Autodesk Inventor part; units mm, degrees
(part 2 of 3)
  line L340 (105.027388, 41.472612) -> (145.027388, 41.472612) construction
  arc A224 (108.377388, 44.822612) -> (108.377388, 38.122612) centre (108.377388, 41.472612) ccw
  arc A225 (91.677388, 38.122612) -> (91.677388, 44.822612) centre (91.677388, 41.472612) ccw
  arc A226 (-58.322612, 38.122612) -> (-58.322612, 44.822612) centre (-58.322612, 41.472612) ccw
  line L341 (-91.622612, 38.122612) -> (-58.322612, 38.122612)
  line L342 (-58.322612, 44.822612) -> (-91.622612, 44.822612)
  line L343 (-94.972612, 41.472612) -> (-54.972612, 41.472612) construction
  arc A227 (-91.622612, 44.822612) -> (-91.622612, 38.122612) centre (-91.622612, 41.472612) ccw
  arc A228 (-41.622612, 34.822612) -> (-41.622612, 28.122612) centre (-41.622612, 31.472612) ccw
  line L344 (-41.622612, 28.122612) -> (-8.322612, 28.122612)
  line L345 (-8.322612, 34.822612) -> (-41.622612, 34.822612)
  line L346 (-44.972612, 31.472612) -> (-4.972612, 31.472612) construction
  arc A229 (-8.322612, 28.122612) -> (-8.322612, 34.822612) centre (-8.322612, 31.472612) ccw
  arc A230 (8.377388, 34.822612) -> (8.377388, 28.122612) centre (8.377388, 31.472612) ccw
  line L347 (8.377388, 28.122612) -> (41.677388, 28.122612)
  line L348 (41.677388, 34.822612) -> (8.377388, 34.822612)
  line L349 (5.027388, 31.472612) -> (45.027388, 31.472612) construction
  arc A231 (58.377388, 34.822612) -> (58.377388, 28.122612) centre (58.377388, 31.472612) ccw
  line L350 (58.377388, 28.122612) -> (91.677388, 28.122612)
  line L351 (91.677388, 34.822612) -> (58.377388, 34.822612)
  line L352 (55.027388, 31.472612) -> (95.027388, 31.472612) construction
  arc A232 (41.677388, 28.122612) -> (41.677388, 34.822612) centre (41.677388, 31.472612) ccw
  arc A233 (158.377388, 34.822612) -> (158.377388, 28.122612) centre (158.377388, 31.472612) ccw
  line L353 (158.377388, 28.122612) -> (191.677388, 28.122612)
  line L354 (191.677388, 34.822612) -> (158.377388, 34.822612)
  line L355 (155.027388, 31.472612) -> (195.027388, 31.472612) construction
  arc A234 (191.677388, 28.122612) -> (191.677388, 34.822612) centre (191.677388, 31.472612) ccw
  arc A235 (141.677388, 28.122612) -> (141.677388, 34.822612) centre (141.677388, 31.472612) ccw
  line L356 (108.377388, 28.122612) -> (141.677388, 28.122612)
  line L357 (141.677388, 34.822612) -> (108.377388, 34.822612)
  line L358 (105.027388, 31.472612) -> (145.027388, 31.472612) construction
  arc A236 (108.377388, 34.822612) -> (108.377388, 28.122612) centre (108.377388, 31.472612) ccw
  arc A237 (91.677388, 28.122612) -> (91.677388, 34.822612) centre (91.677388, 31.472612) ccw
  arc A238 (-58.322612, 28.122612) -> (-58.322612, 34.822612) centre (-58.322612, 31.472612) ccw
  line L359 (-91.622612, 28.122612) -> (-58.322612, 28.122612)
  line L360 (-58.322612, 34.822612) -> (-91.622612, 34.822612)
  line L361 (-94.972612, 31.472612) -> (-54.972612, 31.472612) construction
  arc A239 (-91.622612, 34.822612) -> (-91.622612, 28.122612) centre (-91.622612, 31.472612) ccw
  arc A240 (-41.622612, 24.822612) -> (-41.622612, 18.122612) centre (-41.622612, 21.472612) ccw
  line L362 (-41.622612, 18.122612) -> (-8.322612, 18.122612)
  line L363 (-8.322612, 24.822612) -> (-41.622612, 24.822612)
  line L364 (-44.972612, 21.472612) -> (-4.972612, 21.472612) construction
  arc A241 (-8.322612, 18.122612) -> (-8.322612, 24.822612) centre (-8.322612, 21.472612) ccw
  arc A242 (8.377388, 24.822612) -> (8.377388, 18.122612) centre (8.377388, 21.472612) ccw
  line L365 (8.377388, 18.122612) -> (41.677388, 18.122612)
  line L366 (41.677388, 24.822612) -> (8.377388, 24.822612)
  line L367 (5.027388, 21.472612) -> (45.027388, 21.472612) construction
  arc A243 (58.377388, 24.822612) -> (58.377388, 18.122612) centre (58.377388, 21.472612) ccw
  line L368 (58.377388, 18.122612) -> (91.677388, 18.122612)
  line L369 (91.677388, 24.822612) -> (58.377388, 24.822612)
  line L370 (55.027388, 21.472612) -> (95.027388, 21.472612) construction
  arc A244 (41.677388, 18.122612) -> (41.677388, 24.822612) centre (41.677388, 21.472612) ccw
  arc A245 (158.377388, 24.822612) -> (158.377388, 18.122612) centre (158.377388, 21.472612) ccw
  line L371 (158.377388, 18.122612) -> (191.677388, 18.122612)
  line L372 (191.677388, 24.822612) -> (158.377388, 24.822612)
  line L373 (155.027388, 21.472612) -> (195.027388, 21.472612) construction
  arc A246 (191.677388, 18.122612) -> (191.677388, 24.822612) centre (191.677388, 21.472612) ccw
  arc A247 (141.677388, 18.122612) -> (141.677388, 24.822612) centre (141.677388, 21.472612) ccw
  line L374 (108.377388, 18.122612) -> (141.677388, 18.122612)
  line L375 (141.677388, 24.822612) -> (108.377388, 24.822612)
  line L376 (105.027388, 21.472612) -> (145.027388, 21.472612) construction
  arc A248 (108.377388, 24.822612) -> (108.377388, 18.122612) centre (108.377388, 21.472612) ccw
  arc A249 (91.677388, 18.122612) -> (91.677388, 24.822612) centre (91.677388, 21.472612) ccw
  arc A250 (-58.322612, 18.122612) -> (-58.322612, 24.822612) centre (-58.322612, 21.472612) ccw
  line L377 (-91.622612, 18.122612) -> (-58.322612, 18.122612)
  line L378 (-58.322612, 24.822612) -> (-91.622612, 24.822612)
  line L379 (-94.972612, 21.472612) -> (-54.972612, 21.472612) construction
  arc A251 (-91.622612, 24.822612) -> (-91.622612, 18.122612) centre (-91.622612, 21.472612) ccw
  arc A252 (-41.622612, 14.822612) -> (-41.622612, 8.122612) centre (-41.622612, 11.472612) ccw
  line L380 (-41.622612, 8.122612) -> (-8.322612, 8.122612)
  line L381 (-8.322612, 14.822612) -> (-41.622612, 14.822612)
  line L382 (-44.972612, 11.472612) -> (-4.972612, 11.472612) construction
  arc A253 (-8.322612, 8.122612) -> (-8.322612, 14.822612) centre (-8.322612, 11.472612) ccw
  arc A254 (8.377388, 14.822612) -> (8.377388, 8.122612) centre (8.377388, 11.472612) ccw
  line L383 (8.377388, 8.122612) -> (41.677388, 8.122612)
  line L384 (41.677388, 14.822612) -> (8.377388, 14.822612)
  line L385 (5.027388, 11.472612) -> (45.027388, 11.472612) construction
  arc A255 (58.377388, 14.822612) -> (58.377388, 8.122612) centre (58.377388, 11.472612) ccw
  line L386 (58.377388, 8.122612) -> (91.677388, 8.122612)
  line L387 (91.677388, 14.822612) -> (58.377388, 14.822612)
  line L388 (55.027388, 11.472612) -> (95.027388, 11.472612) construction
  arc A256 (41.677388, 8.122612) -> (41.677388, 14.822612) centre (41.677388, 11.472612) ccw
  arc A257 (158.377388, 14.822612) -> (158.377388, 8.122612) centre (158.377388, 11.472612) ccw
  line L389 (158.377388, 8.122612) -> (191.677388, 8.122612)
  line L390 (191.677388, 14.822612) -> (158.377388, 14.822612)
  line L391 (155.027388, 11.472612) -> (195.027388, 11.472612) construction
  arc A258 (191.677388, 8.122612) -> (191.677388, 14.822612) centre (191.677388, 11.472612) ccw
  arc A259 (141.677388, 8.122612) -> (141.677388, 14.822612) centre (141.677388, 11.472612) ccw
  line L392 (108.377388, 8.122612) -> (141.677388, 8.122612)
  line L393 (141.677388, 14.822612) -> (108.377388, 14.822612)
  line L394 (105.027388, 11.472612) -> (145.027388, 11.472612) construction
  arc A260 (108.377388, 14.822612) -> (108.377388, 8.122612) centre (108.377388, 11.472612) ccw
  arc A261 (91.677388, 8.122612) -> (91.677388, 14.822612) centre (91.677388, 11.472612) ccw
  arc A262 (-58.322612, 8.122612) -> (-58.322612, 14.822612) centre (-58.322612, 11.472612) ccw
  line L395 (-91.622612, 8.122612) -> (-58.322612, 8.122612)
  line L396 (-58.322612, 14.822612) -> (-91.622612, 14.822612)
  line L397 (-94.972612, 11.472612) -> (-54.972612, 11.472612) construction
  arc A263 (-91.622612, 14.822612) -> (-91.622612, 8.122612) centre (-91.622612, 11.472612) ccw
  arc A264 (-41.622612, 4.822612) -> (-41.622612, -1.877388) centre (-41.622612, 1.472612) ccw
  line L398 (-41.622612, -1.877388) -> (-8.322612, -1.877388)
  line L399 (-8.322612, 4.822612) -> (-41.622612, 4.822612)
  line L400 (-44.972612, 1.472612) -> (-4.972612, 1.472612) construction
  arc A265 (-8.322612, -1.877388) -> (-8.322612, 4.822612) centre (-8.322612, 1.472612) ccw
  arc A266 (8.377388, 4.822612) -> (8.377388, -1.877388) centre (8.377388, 1.472612) ccw
  line L401 (8.377388, -1.877388) -> (41.677388, -1.877388)
  line L402 (41.677388, 4.822612) -> (8.377388, 4.822612)
  line L403 (5.027388, 1.472612) -> (45.027388, 1.472612) construction
  arc A267 (58.377388, 4.822612) -> (58.377388, -1.877388) centre (58.377388, 1.472612) ccw
  line L404 (58.377388, -1.877388) -> (91.677388, -1.877388)
  line L405 (91.677388, 4.822612) -> (58.377388, 4.822612)
  line L406 (55.027388, 1.472612) -> (95.027388, 1.472612) construction
  arc A268 (41.677388, -1.877388) -> (41.677388, 4.822612) centre (41.677388, 1.472612) ccw
  arc A269 (158.377388, 4.822612) -> (158.377388, -1.877388) centre (158.377388, 1.472612) ccw
  line L407 (158.377388, -1.877388) -> (191.677388, -1.877388)
  line L408 (191.677388, 4.822612) -> (158.377388, 4.822612)
  line L409 (155.027388, 1.472612) -> (195.027388, 1.472612) construction
  arc A270 (191.677388, -1.877388) -> (191.677388, 4.822612) centre (191.677388, 1.472612) ccw
  arc A271 (141.677388, -1.877388) -> (141.677388, 4.822612) centre (141.677388, 1.472612) ccw
  line L410 (108.377388, -1.877388) -> (141.677388, -1.877388)
  line L411 (141.677388, 4.822612) -> (108.377388, 4.822612)
  line L412 (105.027388, 1.472612) -> (145.027388, 1.472612) construction
  arc A272 (108.377388, 4.822612) -> (108.377388, -1.877388) centre (108.377388, 1.472612) ccw
  arc A273 (91.677388, -1.877388) -> (91.677388, 4.822612) centre (91.677388, 1.472612) ccw
  arc A274 (-58.322612, -1.877388) -> (-58.322612, 4.822612) centre (-58.322612, 1.472612) ccw
  line L413 (-91.622612, -1.877388) -> (-58.322612, -1.877388)
  line L414 (-58.322612, 4.822612) -> (-91.622612, 4.822612)
  line L415 (-94.972612, 1.472612) -> (-54.972612, 1.472612) construction
  arc A275 (-91.622612, 4.822612) -> (-91.622612, -1.877388) centre (-91.622612, 1.472612) ccw
  arc A276 (-41.622612, -5.177388) -> (-41.622612, -11.877388) centre (-41.622612, -8.527388) ccw
  line L416 (-41.622612, -11.877388) -> (-8.322612, -11.877388)
  line L417 (-8.322612, -5.177388) -> (-41.622612, -5.177388)
  line L418 (-44.972612, -8.527388) -> (-4.972612, -8.527388) construction
  arc A277 (-8.322612, -11.877388) -> (-8.322612, -5.177388) centre (-8.322612, -8.527388) ccw
  arc A278 (8.377388, -5.177388) -> (8.377388, -11.877388) centre (8.377388, -8.527388) ccw
  line L419 (8.377388, -11.877388) -> (41.677388, -11.877388)
  line L420 (41.677388, -5.177388) -> (8.377388, -5.177388)
  line L421 (5.027388, -8.527388) -> (45.027388, -8.527388) construction
  arc A279 (58.377388, -5.177388) -> (58.377388, -11.877388) centre (58.377388, -8.527388) ccw
  line L422 (58.377388, -11.877388) -> (91.677388, -11.877388)
  line L423 (91.677388, -5.177388) -> (58.377388, -5.177388)
  line L424 (55.027388, -8.527388) -> (95.027388, -8.527388) construction
  arc A280 (41.677388, -11.877388) -> (41.677388, -5.177388) centre (41.677388, -8.527388) ccw
  arc A281 (158.377388, -5.177388) -> (158.377388, -11.877388) centre (158.377388, -8.527388) ccw
  line L425 (158.377388, -11.877388) -> (191.677388, -11.877388)
  line L426 (191.677388, -5.177388) -> (158.377388, -5.177388)
  line L427 (155.027388, -8.527388) -> (195.027388, -8.527388) construction
  arc A282 (191.677388, -11.877388) -> (191.677388, -5.177388) centre (191.677388, -8.527388) ccw
  arc A283 (141.677388, -11.877388) -> (141.677388, -5.177388) centre (141.677388, -8.527388) ccw
  line L428 (108.377388, -11.877388) -> (141.677388, -11.877388)
  line L429 (141.677388, -5.177388) -> (108.377388, -5.177388)
  line L430 (105.027388, -8.527388) -> (145.027388, -8.527388) construction
  arc A284 (108.377388, -5.177388) -> (108.377388, -11.877388) centre (108.377388, -8.527388) ccw
  arc A285 (91.677388, -11.877388) -> (91.677388, -5.177388) centre (91.677388, -8.527388) ccw
  arc A286 (-58.322612, -11.877388) -> (-58.322612, -5.177388) centre (-58.322612, -8.527388) ccw
  line L431 (-91.622612, -11.877388) -> (-58.322612, -11.877388)
  line L432 (-58.322612, -5.177388) -> (-91.622612, -5.177388)
  line L433 (-94.972612, -8.527388) -> (-54.972612, -8.527388) construction
  arc A287 (-91.622612, -5.177388) -> (-91.622612, -11.877388) centre (-91.622612, -8.527388) ccw
  arc A288 (-41.622612, -15.177388) -> (-41.622612, -21.877388) centre (-41.622612, -18.527388) ccw
  line L434 (-41.622612, -21.877388) -> (-8.322612, -21.877388)
  line L435 (-8.322612, -15.177388) -> (-41.622612, -15.177388)
  line L436 (-44.972612, -18.527388) -> (-4.972612, -18.527388) construction
  arc A289 (-8.322612, -21.877388) -> (-8.322612, -15.177388) centre (-8.322612, -18.527388) ccw
  arc A290 (8.377388, -15.177388) -> (8.377388, -21.877388) centre (8.377388, -18.527388) ccw
  line L437 (8.377388, -21.877388) -> (41.677388, -21.877388)
  line L438 (41.677388, -15.177388) -> (8.377388, -15.177388)
  line L439 (5.027388, -18.527388) -> (45.027388, -18.527388) construction
  arc A291 (58.377388, -15.177388) -> (58.377388, -21.877388) centre (58.377388, -18.527388) ccw
  line L440 (58.377388, -21.877388) -> (91.677388, -21.877388)
  line L441 (91.677388, -15.177388) -> (58.377388, -15.177388)
  line L442 (55.027388, -18.527388) -> (95.027388, -18.527388) construction
  arc A292 (41.677388, -21.877388) -> (41.677388, -15.177388) centre (41.677388, -18.527388) ccw
  arc A293 (158.377388, -15.177388) -> (158.377388, -21.877388) centre (158.377388, -18.527388) ccw
  line L443 (158.377388, -21.877388) -> (191.677388, -21.877388)
  line L444 (191.677388, -15.177388) -> (158.377388, -15.177388)
  line L445 (155.027388, -18.527388) -> (195.027388, -18.527388) construction
  arc A294 (191.677388, -21.877388) -> (191.677388, -15.177388) centre (191.677388, -18.527388) ccw
  arc A295 (141.677388, -21.877388) -> (141.677388, -15.177388) centre (141.677388, -18.527388) ccw
  line L446 (108.377388, -21.877388) -> (141.677388, -21.877388)
  line L447 (141.677388, -15.177388) -> (108.377388, -15.177388)
  line L448 (105.027388, -18.527388) -> (145.027388, -18.527388) construction
  arc A296 (108.377388, -15.177388) -> (108.377388, -21.877388) centre (108.377388, -18.527388) ccw
  arc A297 (91.677388, -21.877388) -> (91.677388, -15.177388) centre (91.677388, -18.527388) ccw
  arc A298 (-58.322612, -21.877388) -> (-58.322612, -15.177388) centre (-58.322612, -18.527388) ccw
  line L449 (-91.622612, -21.877388) -> (-58.322612, -21.877388)
  line L450 (-58.322612, -15.177388) -> (-91.622612, -15.177388)
  line L451 (-94.972612, -18.527388) -> (-54.972612, -18.527388) construction
  arc A299 (-91.622612, -15.177388) -> (-91.622612, -21.877388) centre (-91.622612, -18.527388) ccw
  arc A300 (-41.622612, -25.177388) -> (-41.622612, -31.877388) centre (-41.622612, -28.527388) ccw
  line L452 (-41.622612, -31.877388) -> (-8.322612, -31.877388)
  line L453 (-8.322612, -25.177388) -> (-41.622612, -25.177388)
  line L454 (-44.972612, -28.527388) -> (-4.972612, -28.527388) construction
  arc A301 (-8.322612, -31.877388) -> (-8.322612, -25.177388) centre (-8.322612, -28.527388) ccw
  arc A302 (8.377388, -25.177388) -> (8.377388, -31.877388) centre (8.377388, -28.527388) ccw
  line L455 (8.377388, -31.877388) -> (41.677388, -31.877388)
  line L456 (41.677388, -25.177388) -> (8.377388, -25.177388)
  line L457 (5.027388, -28.527388) -> (45.027388, -28.527388) construction
  arc A303 (58.377388, -25.177388) -> (58.377388, -31.877388) centre (58.377388, -28.527388) ccw
  line L458 (58.377388, -31.877388) -> (91.677388, -31.877388)
  line L459 (91.677388, -25.177388) -> (58.377388, -25.177388)
  line L460 (55.027388, -28.527388) -> (95.027388, -28.527388) construction
  arc A304 (41.677388, -31.877388) -> (41.677388, -25.177388) centre (41.677388, -28.527388) ccw
  arc A305 (158.377388, -25.177388) -> (158.377388, -31.877388) centre (158.377388, -28.527388) ccw
  line L461 (158.377388, -31.877388) -> (191.677388, -31.877388)
  line L462 (191.677388, -25.177388) -> (158.377388, -25.177388)
  line L463 (155.027388, -28.527388) -> (195.027388, -28.527388) construction
  arc A306 (191.677388, -31.877388) -> (191.677388, -25.177388) centre (191.677388, -28.527388) ccw
  arc A307 (141.677388, -31.877388) -> (141.677388, -25.177388) centre (141.677388, -28.527388) ccw
  line L464 (108.377388, -31.877388) -> (141.677388, -31.877388)
  line L465 (141.677388, -25.177388) -> (108.377388, -25.177388)
  line L466 (105.027388, -28.527388) -> (145.027388, -28.527388) construction
  arc A308 (108.377388, -25.177388) -> (108.377388, -31.877388) centre (108.377388, -28.527388) ccw
  arc A309 (91.677388, -31.877388) -> (91.677388, -25.177388) centre (91.677388, -28.527388) ccw
  arc A310 (-58.322612, -31.877388) -> (-58.322612, -25.177388) centre (-58.322612, -28.527388) ccw
  line L467 (-91.622612, -31.877388) -> (-58.322612, -31.877388)
  line L468 (-58.322612, -25.177388) -> (-91.622612, -25.177388)
  line L469 (-94.972612, -28.527388) -> (-54.972612, -28.527388) construction
  arc A311 (-91.622612, -25.177388) -> (-91.622612, -31.877388) centre (-91.622612, -28.527388) ccw
  arc A312 (-41.622612, -35.177388) -> (-41.622612, -41.877388) centre (-41.622612, -38.527388) ccw
  line L470 (-41.622612, -41.877388) -> (-8.322612, -41.877388)
  line L471 (-8.322612, -35.177388) -> (-41.622612, -35.177388)
  line L472 (-44.972612, -38.527388) -> (-4.972612, -38.527388) construction
  arc A313 (-8.322612, -41.877388) -> (-8.322612, -35.177388) centre (-8.322612, -38.527388) ccw
  arc A314 (8.377388, -35.177388) -> (8.377388, -41.877388) centre (8.377388, -38.527388) ccw
  line L473 (8.377388, -41.877388) -> (41.677388, -41.877388)
  line L474 (41.677388, -35.177388) -> (8.377388, -35.177388)
  line L475 (5.027388, -38.527388) -> (45.027388, -38.527388) construction
  arc A315 (58.377388, -35.177388) -> (58.377388, -41.877388) centre (58.377388, -38.527388) ccw
  line L476 (58.377388, -41.877388) -> (91.677388, -41.877388)
  line L477 (91.677388, -35.177388) -> (58.377388, -35.177388)
  line L478 (55.027388, -38.527388) -> (95.027388, -38.527388) construction
  arc A316 (41.677388, -41.877388) -> (41.677388, -35.177388) centre (41.677388, -38.527388) ccw
  arc A317 (158.377388, -35.177388) -> (158.377388, -41.877388) centre (158.377388, -38.527388) ccw
  line L479 (158.377388, -41.877388) -> (191.677388, -41.877388)
  line L480 (191.677388, -35.177388) -> (158.377388, -35.177388)
  line L481 (155.027388, -38.527388) -> (195.027388, -38.527388) construction
  arc A318 (191.677388, -41.877388) -> (191.677388, -35.177388) centre (191.677388, -38.527388) ccw
  arc A319 (141.677388, -41.877388) -> (141.677388, -35.177388) centre (141.677388, -38.527388) ccw
  line L482 (108.377388, -41.877388) -> (141.677388, -41.877388)
  line L483 (141.677388, -35.177388) -> (108.377388, -35.177388)
  line L484 (105.027388, -38.527388) -> (145.027388, -38.527388) construction
  arc A320 (108.377388, -35.177388) -> (108.377388, -41.877388) centre (108.377388, -38.527388) ccw
  arc A321 (91.677388, -41.877388) -> (91.677388, -35.177388) centre (91.677388, -38.527388) ccw
  arc A322 (-58.322612, -41.877388) -> (-58.322612, -35.177388) centre (-58.322612, -38.527388) ccw
  line L485 (-91.622612, -41.877388) -> (-58.322612, -41.877388)
  line L486 (-58.322612, -35.177388) -> (-91.622612, -35.177388)
  line L487 (-94.972612, -38.527388) -> (-54.972612, -38.527388) construction
  arc A323 (-91.622612, -35.177388) -> (-91.622612, -41.877388) centre (-91.622612, -38.527388) ccw
  arc A324 (-41.622612, -45.177388) -> (-41.622612, -51.877388) centre (-41.622612, -48.527388) ccw
  line L488 (-41.622612, -51.877388) -> (-8.322612, -51.877388)
  line L489 (-8.322612, -45.177388) -> (-41.622612, -45.177388)
  line L490 (-44.972612, -48.527388) -> (-4.972612, -48.527388) construction
  arc A325 (-8.322612, -51.877388) -> (-8.322612, -45.177388) centre (-8.322612, -48.527388) ccw
  arc A326 (8.377388, -45.177388) -> (8.377388, -51.877388) centre (8.377388, -48.527388) ccw
  line L491 (8.377388, -51.877388) -> (41.677388, -51.877388)
  line L492 (41.677388, -45.177388) -> (8.377388, -45.177388)
  line L493 (5.027388, -48.527388) -> (45.027388, -48.527388) construction
  arc A327 (58.377388, -45.177388) -> (58.377388, -51.877388) centre (58.377388, -48.527388) ccw
  line L494 (58.377388, -51.877388) -> (91.677388, -51.877388)
  line L495 (91.677388, -45.177388) -> (58.377388, -45.177388)
  line L496 (55.027388, -48.527388) -> (95.027388, -48.527388) construction
  arc A328 (41.677388, -51.877388) -> (41.677388, -45.177388) centre (41.677388, -48.527388) ccw
  arc A329 (158.377388, -45.177388) -> (158.377388, -51.877388) centre (158.377388, -48.527388) ccw
  line L497 (158.377388, -51.877388) -> (191.677388, -51.877388)
  line L498 (191.677388, -45.177388) -> (158.377388, -45.177388)
  line L499 (155.027388, -48.527388) -> (195.027388, -48.527388) construction
  arc A330 (191.677388, -51.877388) -> (191.677388, -45.177388) centre (191.677388, -48.527388) ccw
  arc A331 (141.677388, -51.877388) -> (141.677388, -45.177388) centre (141.677388, -48.527388) ccw
  line L500 (108.377388, -51.877388) -> (141.677388, -51.877388)
  line L501 (141.677388, -45.177388) -> (108.377388, -45.177388)
  line L502 (105.027388, -48.527388) -> (145.027388, -48.527388) construction
  arc A332 (108.377388, -45.177388) -> (108.377388, -51.877388) centre (108.377388, -48.527388) ccw
  arc A333 (91.677388, -51.877388) -> (91.677388, -45.177388) centre (91.677388, -48.527388) ccw
  arc A334 (-58.322612, -51.877388) -> (-58.322612, -45.177388) centre (-58.322612, -48.527388) ccw
  line L503 (-91.622612, -51.877388) -> (-58.322612, -51.877388)
  line L504 (-58.322612, -45.177388) -> (-91.622612, -45.177388)
  line L505 (-94.972612, -48.527388) -> (-54.972612, -48.527388) construction
  arc A335 (-91.622612, -45.177388) -> (-91.622612, -51.877388) centre (-91.622612, -48.527388) ccw
  arc A336 (-41.622612, -55.177388) -> (-41.622612, -61.877388) centre (-41.622612, -58.527388) ccw
  line L506 (-41.622612, -61.877388) -> (-8.322612, -61.877388)
  line L507 (-8.322612, -55.177388) -> (-41.622612, -55.177388)
  line L508 (-44.972612, -58.527388) -> (-4.972612, -58.527388) construction
  arc A337 (-8.322612, -61.877388) -> (-8.322612, -55.177388) centre (-8.322612, -58.527388) ccw
  arc A338 (8.377388, -55.177388) -> (8.377388, -61.877388) centre (8.377388, -58.527388) ccw
  line L509 (8.377388, -61.877388) -> (41.677388, -61.877388)
  line L510 (41.677388, -55.177388) -> (8.377388, -55.177388)
  line L511 (5.027388, -58.527388) -> (45.027388, -58.527388) construction
  arc A339 (58.377388, -55.177388) -> (58.377388, -61.877388) centre (58.377388, -58.527388) ccw
  line L512 (58.377388, -61.877388) -> (91.677388, -61.877388)
  line L513 (91.677388, -55.177388) -> (58.377388, -55.177388)
  line L514 (55.027388, -58.527388) -> (95.027388, -58.527388) construction
  arc A340 (41.677388, -61.877388) -> (41.677388, -55.177388) centre (41.677388, -58.527388) ccw
  arc A341 (158.377388, -55.177388) -> (158.377388, -61.877388) centre (158.377388, -58.527388) ccw
  line L515 (158.377388, -61.877388) -> (191.677388, -61.877388)
  line L516 (191.677388, -55.177388) -> (158.377388, -55.177388)
  line L517 (155.027388, -58.527388) -> (195.027388, -58.527388) construction
  arc A342 (191.677388, -61.877388) -> (191.677388, -55.177388) centre (191.677388, -58.527388) ccw
  arc A343 (141.677388, -61.877388) -> (141.677388, -55.177388) centre (141.677388, -58.527388) ccw
  line L518 (108.377388, -61.877388) -> (141.677388, -61.877388)
  line L519 (141.677388, -55.177388) -> (108.377388, -55.177388)
  line L520 (105.027388, -58.527388) -> (145.027388, -58.527388) construction
  arc A344 (108.377388, -55.177388) -> (108.377388, -61.877388) centre (108.377388, -58.527388) ccw
  arc A345 (91.677388, -61.877388) -> (91.677388, -55.177388) centre (91.677388, -58.527388) ccw
  arc A346 (-58.322612, -61.877388) -> (-58.322612, -55.177388) centre (-58.322612, -58.527388) ccw
  line L521 (-91.622612, -61.877388) -> (-58.322612, -61.877388)
  line L522 (-58.322612, -55.177388) -> (-91.622612, -55.177388)
  line L523 (-94.972612, -58.527388) -> (-54.972612, -58.527388) construction
  arc A347 (-91.622612, -55.177388) -> (-91.622612, -61.877388) centre (-91.622612, -58.527388) ccw
  arc A348 (-41.622612, -65.177388) -> (-41.622612, -71.877388) centre (-41.622612, -68.527388) ccw
  line L524 (-41.622612, -71.877388) -> (-8.322612, -71.877388)
  line L525 (-8.322612, -65.177388) -> (-41.622612, -65.177388)
  line L526 (-44.972612, -68.527388) -> (-4.972612, -68.527388) construction
  arc A349 (-8.322612, -71.877388) -> (-8.322612, -65.177388) centre (-8.322612, -68.527388) ccw
  arc A350 (8.377388, -65.177388) -> (8.377388, -71.877388) centre (8.377388, -68.527388) ccw
  line L527 (8.377388, -71.877388) -> (41.677388, -71.877388)
  line L528 (41.677388, -65.177388) -> (8.377388, -65.177388)
  line L529 (5.027388, -68.527388) -> (45.027388, -68.527388) construction
  arc A351 (58.377388, -65.177388) -> (58.377388, -71.877388) centre (58.377388, -68.527388) ccw
  line L530 (58.377388, -71.877388) -> (91.677388, -71.877388)
  line L531 (91.677388, -65.177388) -> (58.377388, -65.177388)
  line L532 (55.027388, -68.527388) -> (95.027388, -68.527388) construction
  arc A352 (41.677388, -71.877388) -> (41.677388, -65.177388) centre (41.677388, -68.527388) ccw
  arc A353 (158.377388, -65.177388) -> (158.377388, -71.877388) centre (158.377388, -68.527388) ccw
  line L533 (158.377388, -71.877388) -> (191.677388, -71.877388)
  line L534 (191.677388, -65.177388) -> (158.377388, -65.177388)
  line L535 (155.027388, -68.527388) -> (195.027388, -68.527388) construction
  arc A354 (191.677388, -71.877388) -> (191.677388, -65.177388) centre (191.677388, -68.527388) ccw
  arc A355 (141.677388, -71.877388) -> (141.677388, -65.177388) centre (141.677388, -68.527388) ccw
  line L536 (108.377388, -71.877388) -> (141.677388, -71.877388)
  line L537 (141.677388, -65.177388) -> (108.377388, -65.177388)
  line L538 (105.027388, -68.527388) -> (145.027388, -68.527388) construction
  arc A356 (108.377388, -65.177388) -> (108.377388, -71.877388) centre (108.377388, -68.527388) ccw
  arc A357 (91.677388, -71.877388) -> (91.677388, -65.177388) centre (91.677388, -68.527388) ccw
  arc A358 (-58.322612, -71.877388) -> (-58.322612, -65.177388) centre (-58.322612, -68.527388) ccw
  line L539 (-91.622612, -71.877388) -> (-58.322612, -71.877388)
  line L540 (-58.322612, -65.177388) -> (-91.622612, -65.177388)
  line L541 (-94.972612, -68.527388) -> (-54.972612, -68.527388) construction
  arc A359 (-91.622612, -65.177388) -> (-91.622612, -71.877388) centre (-91.622612, -68.527388) ccw
  arc A360 (-41.622612, -75.177388) -> (-41.622612, -81.877388) centre (-41.622612, -78.527388) ccw
  line L542 (-41.622612, -81.877388) -> (-8.322612, -81.877388)
  line L543 (-8.322612, -75.177388) -> (-41.622612, -75.177388)
  line L544 (-44.972612, -78.527388) -> (-4.972612, -78.527388) construction
  arc A361 (-8.322612, -81.877388) -> (-8.322612, -75.177388) centre (-8.322612, -78.527388) ccw
  arc A362 (8.377388, -75.177388) -> (8.377388, -81.877388) centre (8.377388, -78.527388) ccw
  line L545 (8.377388, -81.877388) -> (41.677388, -81.877388)
  line L546 (41.677388, -75.177388) -> (8.377388, -75.177388)
  line L547 (5.027388, -78.527388) -> (45.027388, -78.527388) construction
  arc A363 (58.377388, -75.177388) -> (58.377388, -81.877388) centre (58.377388, -78.527388) ccw
  line L548 (58.377388, -81.877388) -> (91.677388, -81.877388)
  line L549 (91.677388, -75.177388) -> (58.377388, -75.177388)
  line L550 (55.027388, -78.527388) -> (95.027388, -78.527388) construction
  arc A364 (41.677388, -81.877388) -> (41.677388, -75.177388) centre (41.677388, -78.527388) ccw
  arc A365 (158.377388, -75.177388) -> (158.377388, -81.877388) centre (158.377388, -78.527388) ccw
  line L551 (158.377388, -81.877388) -> (191.677388, -81.877388)
  line L552 (191.677388, -75.177388) -> (158.377388, -75.177388)
  line L553 (155.027388, -78.527388) -> (195.027388, -78.527388) construction
  arc A366 (191.677388, -81.877388) -> (191.677388, -75.177388) centre (191.677388, -78.527388) ccw
  arc A367 (141.677388, -81.877388) -> (141.677388, -75.177388) centre (141.677388, -78.527388) ccw
  line L554 (108.377388, -81.877388) -> (141.677388, -81.877388)
  line L555 (141.677388, -75.177388) -> (108.377388, -75.177388)
  line L556 (105.027388, -78.527388) -> (145.027388, -78.527388) construction
  arc A368 (108.377388, -75.177388) -> (108.377388, -81.877388) centre (108.377388, -78.527388) ccw
  arc A369 (91.677388, -81.877388) -> (91.677388, -75.177388) centre (91.677388, -78.527388) ccw
  arc A370 (-58.322612, -81.877388) -> (-58.322612, -75.177388) centre (-58.322612, -78.527388) ccw
  line L557 (-91.622612, -81.877388) -> (-58.322612, -81.877388)
  line L558 (-58.322612, -75.177388) -> (-91.622612, -75.177388)
  line L559 (-94.972612, -78.527388) -> (-54.972612, -78.527388) construction
  arc A371 (-91.622612, -75.177388) -> (-91.622612, -81.877388) centre (-91.622612, -78.527388) ccw
  arc A372 (-41.622612, -85.177388) -> (-41.622612, -91.877388) centre (-41.622612, -88.527388) ccw
  line L560 (-41.622612, -91.877388) -> (-8.322612, -91.877388)
  line L561 (-8.322612, -85.177388) -> (-41.622612, -85.177388)
  line L562 (-44.972612, -88.527388) -> (-4.972612, -88.527388) construction
  arc A373 (-8.322612, -91.877388) -> (-8.322612, -85.177388) centre (-8.322612, -88.527388) ccw
  arc A374 (8.377388, -85.177388) -> (8.377388, -91.877388) centre (8.377388, -88.527388) ccw
  line L563 (8.377388, -91.877388) -> (41.677388, -91.877388)
  line L564 (41.677388, -85.177388) -> (8.377388, -85.177388)
  line L565 (5.027388, -88.527388) -> (45.027388, -88.527388) construction
  arc A375 (58.377388, -85.177388) -> (58.377388, -91.877388) centre (58.377388, -88.527388) ccw
  line L566 (58.377388, -91.877388) -> (91.677388, -91.877388)
  line L567 (91.677388, -85.177388) -> (58.377388, -85.177388)
  line L568 (55.027388, -88.527388) -> (95.027388, -88.527388) construction
  arc A376 (41.677388, -91.877388) -> (41.677388, -85.177388) centre (41.677388, -88.527388) ccw
  arc A377 (158.377388, -85.177388) -> (158.377388, -91.877388) centre (158.377388, -88.527388) ccw
  line L569 (158.377388, -91.877388) -> (191.677388, -91.877388)
  line L570 (191.677388, -85.177388) -> (158.377388, -85.177388)
  line L571 (155.027388, -88.527388) -> (195.027388, -88.527388) construction
  arc A378 (191.677388, -91.877388) -> (191.677388, -85.177388) centre (191.677388, -88.527388) ccw
  arc A379 (141.677388, -91.877388) -> (141.677388, -85.177388) centre (141.677388, -88.527388) ccw
  line L572 (108.377388, -91.877388) -> (141.677388, -91.877388)
  line L573 (141.677388, -85.177388) -> (108.377388, -85.177388)
  line L574 (105.027388, -88.527388) -> (145.027388, -88.527388) construction
  arc A380 (108.377388, -85.177388) -> (108.377388, -91.877388) centre (108.377388, -88.527388) ccw
  arc A381 (91.677388, -91.877388) -> (91.677388, -85.177388) centre (91.677388, -88.527388) ccw
  arc A382 (-58.322612, -91.877388) -> (-58.322612, -85.177388) centre (-58.322612, -88.527388) ccw
  line L575 (-91.622612, -91.877388) -> (-58.322612, -91.877388)
  line L576 (-58.322612, -85.177388) -> (-91.622612, -85.177388)
  line L577 (-94.972612, -88.527388) -> (-54.972612, -88.527388) construction
  arc A383 (-91.622612, -85.177388) -> (-91.622612, -91.877388) centre (-91.622612, -88.527388) ccw
  arc A384 (-41.622612, -95.177388) -> (-41.622612, -101.877388) centre (-41.622612, -98.527388) ccw
  line L578 (-41.622612, -101.877388) -> (-8.322612, -101.877388)
  line L579 (-8.322612, -95.177388) -> (-41.622612, -95.177388)
  line L580 (-44.972612, -98.527388) -> (-4.972612, -98.527388) construction
  arc A385 (-8.322612, -101.877388) -> (-8.322612, -95.177388) centre (-8.322612, -98.527388) ccw
  arc A386 (8.377388, -95.177388) -> (8.377388, -101.877388) centre (8.377388, -98.527388) ccw
  line L581 (8.377388, -101.877388) -> (41.677388, -101.877388)
  line L582 (41.677388, -95.177388) -> (8.377388, -95.177388)
  line L583 (5.027388, -98.527388) -> (45.027388, -98.527388) construction
  arc A387 (58.377388, -95.177388) -> (58.377388, -101.877388) centre (58.377388, -98.527388) ccw
  line L584 (58.377388, -101.877388) -> (91.677388, -101.877388)
  line L585 (91.677388, -95.177388) -> (58.377388, -95.177388)
  line L586 (55.027388, -98.527388) -> (95.027388, -98.527388) construction
  arc A388 (41.677388, -101.877388) -> (41.677388, -95.177388) centre (41.677388, -98.527388) ccw
  arc A389 (158.377388, -95.177388) -> (158.377388, -101.877388) centre (158.377388, -98.527388) ccw
  line L587 (158.377388, -101.877388) -> (191.677388, -101.877388)
  line L588 (191.677388, -95.177388) -> (158.377388, -95.177388)
  line L589 (155.027388, -98.527388) -> (195.027388, -98.527388) construction
  arc A390 (191.677388, -101.877388) -> (191.677388, -95.177388) centre (191.677388, -98.527388) ccw
  arc A391 (141.677388, -101.877388) -> (141.677388, -95.177388) centre (141.677388, -98.527388) ccw
  line L590 (108.377388, -101.877388) -> (141.677388, -101.877388)
  line L591 (141.677388, -95.177388) -> (108.377388, -95.177388)
  line L592 (105.027388, -98.527388) -> (145.027388, -98.527388) construction
  arc A392 (108.377388, -95.177388) -> (108.377388, -101.877388) centre (108.377388, -98.527388) ccw
  arc A393 (91.677388, -101.877388) -> (91.677388, -95.177388) centre (91.677388, -98.527388) ccw
  arc A394 (-58.322612, -101.877388) -> (-58.322612, -95.177388) centre (-58.322612, -98.527388) ccw
  line L593 (-91.622612, -101.877388) -> (-58.322612, -101.877388)
  line L594 (-58.322612, -95.177388) -> (-91.622612, -95.177388)
  line L595 (-94.972612, -98.527388) -> (-54.972612, -98.527388) construction
  arc A395 (-91.622612, -95.177388) -> (-91.622612, -101.877388) centre (-91.622612, -98.527388) ccw
  arc A396 (-41.622612, -105.177388) -> (-41.622612, -111.877388) centre (-41.622612, -108.527388) ccw
  line L596 (-41.622612, -111.877388) -> (-8.322612, -111.877388)
  line L597 (-8.322612, -105.177388) -> (-41.622612, -105.177388)
  line L598 (-44.972612, -108.527388) -> (-4.972612, -108.527388) construction
  arc A397 (-8.322612, -111.877388) -> (-8.322612, -105.177388) centre (-8.322612, -108.527388) ccw
  arc A398 (8.377388, -105.177388) -> (8.377388, -111.877388) centre (8.377388, -108.527388) ccw
  line L599 (8.377388, -111.877388) -> (41.677388, -111.877388)
  line L600 (41.677388, -105.177388) -> (8.377388, -105.177388)
  line L601 (5.027388, -108.527388) -> (45.027388, -108.527388) construction
  arc A399 (58.377388, -105.177388) -> (58.377388, -111.877388) centre (58.377388, -108.527388) ccw
  line L602 (58.377388, -111.877388) -> (91.677388, -111.877388)
  line L603 (91.677388, -105.177388) -> (58.377388, -105.177388)
  line L604 (55.027388, -108.527388) -> (95.027388, -108.527388) construction
  arc A400 (41.677388, -111.877388) -> (41.677388, -105.177388) centre (41.677388, -108.527388) ccw
  arc A401 (158.377388, -105.177388) -> (158.377388, -111.877388) centre (158.377388, -108.527388) ccw
  line L605 (158.377388, -111.877388) -> (191.677388, -111.877388)
  line L606 (191.677388, -105.177388) -> (158.377388, -105.177388)
  line L607 (155.027388, -108.527388) -> (195.027388, -108.527388) construction
  arc A402 (191.677388, -111.877388) -> (191.677388, -105.177388) centre (191.677388, -108.527388) ccw
  arc A403 (141.677388, -111.877388) -> (141.677388, -105.177388) centre (141.677388, -108.527388) ccw
  line L608 (108.377388, -111.877388) -> (141.677388, -111.877388)
  line L609 (141.677388, -105.177388) -> (108.377388, -105.177388)
  line L610 (105.027388, -108.527388) -> (145.027388, -108.527388) construction
  arc A404 (108.377388, -105.177388) -> (108.377388, -111.877388) centre (108.377388, -108.527388) ccw
  arc A405 (91.677388, -111.877388) -> (91.677388, -105.177388) centre (91.677388, -108.527388) ccw
  arc A406 (-58.322612, -111.877388) -> (-58.322612, -105.177388) centre (-58.322612, -108.527388) ccw
  line L611 (-91.622612, -111.877388) -> (-58.322612, -111.877388)
  line L612 (-58.322612, -105.177388) -> (-91.622612, -105.177388)
  line L613 (-94.972612, -108.527388) -> (-54.972612, -108.527388) construction
  arc A407 (-91.622612, -105.177388) -> (-91.622612, -111.877388) centre (-91.622612, -108.527388) ccw
  arc A408 (-41.622612, -115.177388) -> (-41.622612, -121.877388) centre (-41.622612, -118.527388) ccw
  line L614 (-41.622612, -121.877388) -> (-8.322612, -121.877388)
  line L615 (-8.322612, -115.177388) -> (-41.622612, -115.177388)
  line L616 (-44.972612, -118.527388) -> (-4.972612, -118.527388) construction
  arc A409 (-8.322612, -121.877388) -> (-8.322612, -115.177388) centre (-8.322612, -118.527388) ccw
  arc A410 (8.377388, -115.177388) -> (8.377388, -121.877388) centre (8.377388, -118.527388) ccw
  line L617 (8.377388, -121.877388) -> (41.677388, -121.877388)
  line L618 (41.677388, -115.177388) -> (8.377388, -115.177388)
  line L619 (5.027388, -118.527388) -> (45.027388, -118.527388) construction
  arc A411 (58.377388, -115.177388) -> (58.377388, -121.877388) centre (58.377388, -118.527388) ccw
  line L620 (58.377388, -121.877388) -> (91.677388, -121.877388)
  line L621 (91.677388, -115.177388) -> (58.377388, -115.177388)
  line L622 (55.027388, -118.527388) -> (95.027388, -118.527388) construction
  arc A412 (41.677388, -121.877388) -> (41.677388, -115.177388) centre (41.677388, -118.527388) ccw
  arc A413 (158.377388, -115.177388) -> (158.377388, -121.877388) centre (158.377388, -118.527388) ccw
  line L623 (158.377388, -121.877388) -> (191.677388, -121.877388)
  line L624 (191.677388, -115.177388) -> (158.377388, -115.177388)
  line L625 (155.027388, -118.527388) -> (195.027388, -118.527388) construction
  arc A414 (191.677388, -121.877388) -> (191.677388, -115.177388) centre (191.677388, -118.527388) ccw
  arc A415 (141.677388, -121.877388) -> (141.677388, -115.177388) centre (141.677388, -118.527388) ccw
  line L626 (108.377388, -121.877388) -> (141.677388, -121.877388)
  line L627 (141.677388, -115.177388) -> (108.377388, -115.177388)
  line L628 (105.027388, -118.527388) -> (145.027388, -118.527388) construction
  arc A416 (108.377388, -115.177388) -> (108.377388, -121.877388) centre (108.377388, -118.527388) ccw
  arc A417 (91.677388, -121.877388) -> (91.677388, -115.177388) centre (91.677388, -118.527388) ccw
  arc A418 (-58.322612, -121.877388) -> (-58.322612, -115.177388) centre (-58.322612, -118.527388) ccw
  line L629 (-91.622612, -121.877388) -> (-58.322612, -121.877388)
  line L630 (-58.322612, -115.177388) -> (-91.622612, -115.177388)
  line L631 (-94.972612, -118.527388) -> (-54.972612, -118.527388) construction
  arc A419 (-91.622612, -115.177388) -> (-91.622612, -121.877388) centre (-91.622612, -118.527388) ccw
  arc A420 (-41.622612, -125.177388) -> (-41.622612, -131.877388) centre (-41.622612, -128.527388) ccw
  line L632 (-41.622612, -131.877388) -> (-8.322612, -131.877388)
  line L633 (-8.322612, -125.177388) -> (-41.622612, -125.177388)
  line L634 (-44.972612, -128.527388) -> (-4.972612, -128.527388) construction
  arc A421 (-8.322612, -131.877388) -> (-8.322612, -125.177388) centre (-8.322612, -128.527388) ccw
  arc A422 (8.377388, -125.177388) -> (8.377388, -131.877388) centre (8.377388, -128.527388) ccw
  line L635 (8.377388, -131.877388) -> (41.677388, -131.877388)
  line L636 (41.677388, -125.177388) -> (8.377388, -125.177388)
  line L637 (5.027388, -128.527388) -> (45.027388, -128.527388) construction
  arc A423 (58.377388, -125.177388) -> (58.377388, -131.877388) centre (58.377388, -128.527388) ccw
  line L638 (58.377388, -131.877388) -> (91.677388, -131.877388)
  line L639 (91.677388, -125.177388) -> (58.377388, -125.177388)
  line L640 (55.027388, -128.527388) -> (95.027388, -128.527388) construction
  arc A424 (41.677388, -131.877388) -> (41.677388, -125.177388) centre (41.677388, -128.527388) ccw
  arc A425 (158.377388, -125.177388) -> (158.377388, -131.877388) centre (158.377388, -128.527388) ccw
  line L641 (158.377388, -131.877388) -> (191.677388, -131.877388)
  line L642 (191.677388, -125.177388) -> (158.377388, -125.177388)
  line L643 (155.027388, -128.527388) -> (195.027388, -128.527388) construction
  arc A426 (191.677388, -131.877388) -> (191.677388, -125.177388) centre (191.677388, -128.527388) ccw
  arc A427 (141.677388, -131.877388) -> (141.677388, -125.177388) centre (141.677388, -128.527388) ccw
  line L644 (108.377388, -131.877388) -> (141.677388, -131.877388)
  line L645 (141.677388, -125.177388) -> (108.377388, -125.177388)
  line L646 (105.027388, -128.527388) -> (145.027388, -128.527388) construction
  arc A428 (108.377388, -125.177388) -> (108.377388, -131.877388) centre (108.377388, -128.527388) ccw
  arc A429 (91.677388, -131.877388) -> (91.677388, -125.177388) centre (91.677388, -128.527388) ccw
  arc A430 (-58.322612, -131.877388) -> (-58.322612, -125.177388) centre (-58.322612, -128.527388) ccw
  line L647 (-91.622612, -131.877388) -> (-58.322612, -131.877388)
  line L648 (-58.322612, -125.177388) -> (-91.622612, -125.177388)
  line L649 (-94.972612, -128.527388) -> (-54.972612, -128.527388) construction
  arc A431 (-91.622612, -125.177388) -> (-91.622612, -131.877388) centre (-91.622612, -128.527388) ccw
  point P0 (0, 0)
  point P1 (-174.972612, 131.472612)
  point P2 (-124.972612, 131.472612)
  point P3 (-74.972612, 131.472612)
  point P4 (-24.972612, 131.472612)
  point P5 (25.027388, 131.472612)
  point P6 (75.027388, 131.472612)
  point P7 (125.027388, 131.472612)
  point P8 (175.027388, 131.472612)
  point P9 (-174.972612, 121.472612)
  point P10 (-174.972612, 111.472612)
  point P11 (-174.972612, 101.472612)
  point P12 (-174.972612, 91.472612)
  point P13 (-174.972612, 81.472612)
  point P14 (-174.972612, 71.472612)
  point P15 (-174.972612, 61.472612)
  point P16 (-174.972612, 51.472612)
  point P17 (-174.972612, 41.472612)
  point P18 (-174.972612, 31.472612)
  point P19 (-174.972612, 21.472612)
  point P20 (-174.972612, 11.472612)
  point P21 (-174.972612, 1.472612)
  point P22 (-174.972612, -8.527388)
  point P23 (-174.972612, -18.527388)
  point P24 (-174.972612, -28.527388)
  point P25 (-174.972612, -38.527388)
  point P26 (-174.972612, -48.527388)
  point P27 (-174.972612, -58.527388)
  point P28 (-174.972612, -68.527388)
  point P29 (-174.972612, -78.527388)
  point P30 (-174.972612, -88.527388)
  point P31 (-174.972612, -98.527388)
  point P32 (-174.972612, -108.527388)
  point P33 (-174.972612, -118.527388)
  point P34 (-174.972612, -128.527388)
  point P35 (-124.972612, 121.472612)
  point P36 (-124.972612, 111.472612)
  point P37 (-124.972612, 101.472612)
  point P38 (-124.972612, 91.472612)
  point P39 (-124.972612, 81.472612)
  point P40 (-124.972612, 71.472612)
  point P41 (-124.972612, 61.472612)
  point P42 (-124.972612, 51.472612)
  point P43 (-124.972612, 41.472612)
  point P44 (-124.972612, 31.472612)
  point P45 (-124.972612, 21.472612)
  point P46 (-124.972612, 11.472612)
  point P47 (-124.972612, 1.472612)
  point P48 (-124.972612, -8.527388)
  point P49 (-124.972612, -18.527388)
  point P50 (-124.972612, -28.527388)
  point P51 (-124.972612, -38.527388)
  point P52 (-124.972612, -48.527388)
  point P53 (-124.972612, -58.527388)
  point P54 (-124.972612, -68.527388)
  point P55 (-124.972612, -78.527388)
  point P56 (-124.972612, -88.527388)
  point P57 (-124.972612, -98.527388)
  point P58 (-124.972612, -108.527388)
  point P59 (-124.972612, -118.527388)
  point P60 (-124.972612, -128.527388)
  point P61 (-24.972612, 121.472612)
  point P62 (25.027388, 121.472612)
  point P63 (75.027388, 121.472612)
  point P64 (175.027388, 121.472612)
  point P65 (125.027388, 121.472612)
  point P66 (-74.972612, 121.472612)
  point P67 (-24.972612, 111.472612)
  point P68 (25.027388, 111.472612)
  point P69 (75.027388, 111.472612)
  point P70 (175.027388, 111.472612)
  point P71 (125.027388, 111.472612)
  point P72 (-74.972612, 111.472612)
  point P73 (-24.972612, 101.472612)
  point P74 (25.027388, 101.472612)
  point P75 (75.027388, 101.472612)
  point P76 (175.027388, 101.472612)
  point P77 (125.027388, 101.472612)
  point P78 (-74.972612, 101.472612)
  point P79 (-24.972612, 91.472612)
  point P80 (25.027388, 91.472612)
  point P81 (75.027388, 91.472612)
  point P82 (175.027388, 91.472612)
  point P83 (125.027388, 91.472612)
  point P84 (-74.972612, 91.472612)
  point P85 (-24.972612, 81.472612)
  point P86 (25.027388, 81.472612)
  point P87 (75.027388, 81.472612)
  point P88 (175.027388, 81.472612)
  point P89 (125.027388, 81.472612)
  point P90 (-74.972612, 81.472612)
  point P91 (-24.972612, 71.472612)
  point P92 (25.027388, 71.472612)
  point P93 (75.027388, 71.472612)
  point P94 (175.027388, 71.472612)
  point P95 (125.027388, 71.472612)
  point P96 (-74.972612, 71.472612)
  point P97 (-24.972612, 61.472612)
  point P98 (25.027388, 61.472612)
  point P99 (75.027388, 61.472612)
  point P100 (175.027388, 61.472612)
  point P101 (125.027388, 61.472612)
  point P102 (-74.972612, 61.472612)
  point P103 (-24.972612, 51.472612)
  point P104 (25.027388, 51.472612)
  point P105 (75.027388, 51.472612)
  point P106 (175.027388, 51.472612)
  point P107 (125.027388, 51.472612)
  point P108 (-74.972612, 51.472612)
  point P109 (-24.972612, 41.472612)
  point P110 (25.027388, 41.472612)
  point P111 (75.027388, 41.472612)
  point P112 (175.027388, 41.472612)
  point P113 (125.027388, 41.472612)
  point P114 (-74.972612, 41.472612)
  point P115 (-24.972612, 31.472612)
  point P116 (25.027388, 31.472612)
  point P117 (75.027388, 31.472612)
  point P118 (175.027388, 31.472612)
  point P119 (125.027388, 31.472612)
  point P120 (-74.972612, 31.472612)
  point P121 (-24.972612, 21.472612)
  point P122 (25.027388, 21.472612)
  point P123 (75.027388, 21.472612)
  point P124 (175.027388, 21.472612)
  point P125 (125.027388, 21.472612)
  point P126 (-74.972612, 21.472612)
  point P127 (-24.972612, 11.472612)
  point P128 (25.027388, 11.472612)
  point P129 (75.027388, 11.472612)
  point P130 (175.027388, 11.472612)
  point P131 (125.027388, 11.472612)
  point P132 (-74.972612, 11.472612)
  point P133 (-24.972612, 1.472612)
  point P134 (25.027388, 1.472612)
  point P135 (75.027388, 1.472612)
  point P136 (175.027388, 1.472612)
  point P137 (125.027388, 1.472612)
  point P138 (-74.972612, 1.472612)
  point P139 (-24.972612, -8.527388)
  point P140 (25.027388, -8.527388)
  point P141 (75.027388, -8.527388)
  point P142 (175.027388, -8.527388)
  point P143 (125.027388, -8.527388)
  point P144 (-74.972612, -8.527388)
  point P145 (-24.972612, -18.527388)
  point P146 (25.027388, -18.527388)
  point P147 (75.027388, -18.527388)
  point P148 (175.027388, -18.527388)
  point P149 (125.027388, -18.527388)
  point P150 (-74.972612, -18.527388)
  point P151 (-24.972612, -28.527388)
  point P152 (25.027388, -28.527388)
  point P153 (75.027388, -28.527388)
  point P154 (175.027388, -28.527388)
  point P155 (125.027388, -28.527388)
  point P156 (-74.972612, -28.527388)
  point P157 (-24.972612, -38.527388)
  point P158 (25.027388, -38.527388)
  point P159 (75.027388, -38.527388)
  point P160 (175.027388, -38.527388)
  point P161 (125.027388, -38.527388)
  point P162 (-74.972612, -38.527388)
  point P163 (-24.972612, -48.527388)
  point P164 (25.027388, -48.527388)
  point P165 (75.027388, -48.527388)
  point P166 (175.027388, -48.527388)
  point P167 (125.027388, -48.527388)
  point P168 (-74.972612, -48.527388)
  point P169 (-24.972612, -58.527388)
  point P170 (25.027388, -58.527388)
  point P171 (75.027388, -58.527388)
  point P172 (175.027388, -58.527388)
  point P173 (125.027388, -58.527388)
  point P174 (-74.972612, -58.527388)
  point P175 (-24.972612, -68.527388)
  point P176 (25.027388, -68.527388)
  point P177 (75.027388, -68.527388)
  point P178 (175.027388, -68.527388)
  point P179 (125.027388, -68.527388)
  point P180 (-74.972612, -68.527388)
  point P181 (-24.972612, -78.527388)
  point P182 (25.027388, -78.527388)
  point P183 (75.027388, -78.527388)
  point P184 (175.027388, -78.527388)
  point P185 (125.027388, -78.527388)
  point P186 (-74.972612, -78.527388)
  point P187 (-24.972612, -88.527388)
  point P188 (25.027388, -88.527388)
  point P189 (75.027388, -88.527388)
  point P190 (175.027388, -88.527388)
  point P191 (125.027388, -88.527388)
  point P192 (-74.972612, -88.527388)
  point P193 (-24.972612, -98.527388)
  point P194 (25.027388, -98.527388)
  point P195 (75.027388, -98.527388)
  point P196 (175.027388, -98.527388)
  point P197 (125.027388, -98.527388)
  point P198 (-74.972612, -98.527388)
  point P199 (-24.972612, -108.527388)
  dimension "d12" = 40
  dimension "d13" = 6.7
  dimension "d14" = 8.5
  dimension "d17" = 50
  dimension "d22" = 7
  dimension "d25" = 10
  dimension "d32" = 10
  dimension "d39" = 10
  constraints: 1728 end point, 1296 point on circle, 432 centre point, 432 point on line, 4 tangent, 3 vertical, 2 horizontal, 1 midpoint, 1 parallel, 3010 other
  measures "d12" distance of L0.start L0.end
  measures "d13" diameter of A1
  measures "d14" distance from line of L3 L0.start
  measures "d17" distance of L1.start L6.start
  measures "d22" distance from line of L4 point (-174.973, 131.473)
  measures "d25" distance of L1.start L26.start
  measures "d32" distance of L6.start L104.start
  measures "d39" distance of L11.start L184.start
extrude "Extrusión3" cut sketch "Boceto6" against normal blind 2